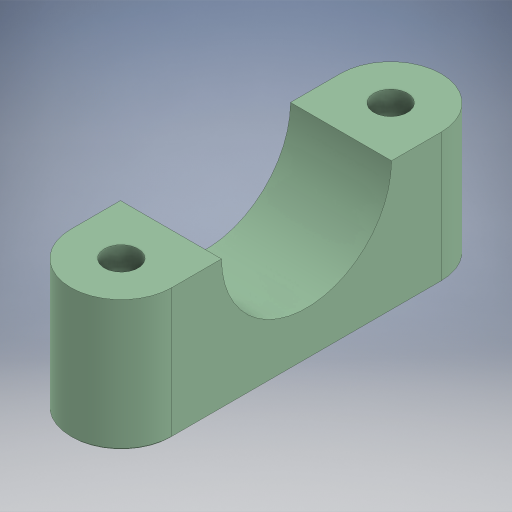
# Autodesk Inventor part: motor_mount_edge_part2
Saved by Autodesk Inventor 2023 (Build 270158000, 158)
## iProperties
Created: 2024-09-12
Part Number: motor_mount_edge_part2
Material: Полиэтилен, низкая плотность
Document SubType Name: Modeling
Designer: Ivan
Density: 0.894 g/cm^3
Appearance: Резина — зеленая
Mass: 4.68214 g
Surface Area: 27.073 cm^2
Volume: 5.23729 cm^3
Высота_крепления: 15,500 мм
Диаметр_мотора: 20,200 мм
d0: 15,000 мм
d1: 44,000 мм
d2: 16,000 мм
d3: 4,000 мм
d5: 0,00 град
d8: 0,00 град
Author: Ivan
Autodesk Inventor part; units mm, degrees
ref_plane "YZ Plane" through (0, 0, 0) normal (1, 0, 0) x (0, 1, 0)
ref_plane "XZ Plane" through (0, 0, 0) normal (0, 1, 0) x (-1, 0, 0)
ref_plane "XY Plane" through (0, 0, 0) normal (0, 0, 1) x (1, 0, 0)
sketch "Эскиз1" plane through (0, 0, 0) normal (0, 1, 0) x (-1, 0, 0)
  line L0 (7.5, 22) -> (-7.5, 22)
  line L1 (-7.5, 22) -> (-7.5, -22)
  line L2 (-7.5, -22) -> (7.5, -22)
  line L3 (7.5, -22) -> (7.5, 22)
  line L4 (-7.5, 22) -> (7.5, -22) construction
  line L5 (0, 22) -> (0, -22) construction
  circle A0 centre (0, 16) radius 2
  line L6 (7.5, 0) -> (-7.5, 0) construction
  circle A1 centre (0, -16) radius 2
  point P0 (0, 0)
  point P1 (0, 0)
  dimension "d0" = 15
  dimension "d1" = 44
  dimension "d2" = 16
  dimension "d3" = 4
  constraints: 14 end point, 5 midpoint, 2 centre point, 2 coincident, 2 parallel, 1 horizontal, 1 perpendicular, 1 point on line, 1 symmetric about line, 1 other
  measures "d0" distance of L2.end L1.end
  measures "d1" distance of L0.end L1.end
  measures "d2" distance of point (0, 0) point (0, 16)
  measures "d3" diameter of A0
extrude "Выдавливание1" add sketch "Эскиз1" along normal blind 15.5
sketch "Эскиз2" plane through (7.5, 0, 22) normal (1, 0, 0) x (0, 0, -1)
  line L0 (0, 15.5) -> (44, 15.5) projected
  circle A0 centre (22, 15.5) radius 10.1
  point P0 (22, 0)
  dimension "Диаметр_мотора" = 20.2
  constraints: 1 centre point, 1 midpoint
  measures "Диаметр_мотора" diameter of A0
extrude "Выдавливание2" cut sketch "Эскиз2" against normal through all
sketch "Эскиз4" plane through (0, 15.5, 0) normal (0, 1, 0) x (1, 0, 0)
  circle A0 centre (0, 16) radius 3.5
  circle A1 centre (0, 16) radius 2 projected
  line L0 (-6, 12.5) -> (6, 12.5)
  line L1 (6, 16) -> (6, 0)
  line L2 (6, 0) -> (-6, 0)
  line L3 (-6, 0) -> (-6, 16)
  line L4 (-6, 12.5) -> (6, 0) construction
  line L5 (0, 0) -> (0, 16) construction
  arc A2 (6, 16) -> (-6, 16) centre (0, 16) ccw
  line L6 (7.5, 22) -> (-7.5, 22) projected
  line L7 (6, -16) -> (6, 0)
  line L8 (-6, 0) -> (-6, -16)
  arc A3 (-6, -16) -> (6, -16) centre (0, -16) ccw
  line L9 (7.5, 22) -> (-7.5, 22) projected
  line L10 (7.5, -22) -> (7.5, 22) projected
  line L11 (-7.5, 22) -> (7.5, 22)
  line L12 (7.5, 22) -> (7.5, -22)
  line L13 (7.5, -22) -> (-7.5, -22)
  line L14 (-7.5, -22) -> (-7.5, 22)
  point P0 (0, 6.25)
  point P1 (0, 12.5)
  point P2 (0, 22)
  point P3 (0, -22)
  dimension "d12" = 7
  constraints: 24 end point, 5 point on circle, 4 midpoint, 4 parallel, 3 point on line, 3 symmetric about line, 2 centre point, 2 coincident, 2 horizontal, 2 perpendicular, 1 vertical, 1 vertical alignment, 3 other
extrude "Выдавливание3" cut sketch "Эскиз4" against normal through all contours L3 L8 A3 L13 L14 L6 A2 | L1 A2 L6 L10 L13 A3 L7
chamfer "Фаска2" distance 0.2 angle 45 6 edges at (0, 0, 22) (-6, 0, 0) (0, 0, -22) (6, 0, 0) (2, 0, 16) (2, 0, -16)
